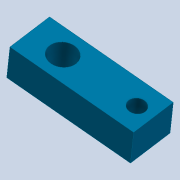
# Autodesk Inventor part: Part3_slider
Saved by Autodesk Inventor 2020 (Build 240168000, 168)
## iProperties
Created: 2019-05-16
Part Number: Part3_slider
Material: ABS Plastic
Document SubType Name: Modeling
Designer: kimhos
Density: 1.06 g/cm^3
Appearance: Sky Blue Medium
Author: kimhos
Autodesk Inventor part; units mm, degrees
ref_plane "YZ Plane" through (0, 0, 0) normal (1, 0, 0) x (0, 1, 0)
ref_plane "XZ Plane" through (0, 0, 0) normal (0, 1, 0) x (-1, 0, 0)
ref_plane "XY Plane" through (0, 0, 0) normal (0, 0, 1) x (1, 0, 0)
sketch "Sketch2" plane through (0, 0, 0) normal (0, 1, 0) x (-1, 0, 0)
  line L0 (1.35, 0) -> (1.35, -4.5)
  line L1 (-1.35, -1) -> (-1.35, 3)
  line L2 (-1.35, -4.5) -> (-1.35, 3)
  line L3 (-1.35, 3) -> (1.35, 3)
  line L4 (1.35, 3) -> (1.35, -4.5)
  line L5 (-1.35, -4.5) -> (1.35, -4.5)
  point P0 (0, 0)
  dimension "d8" = 1.35
  dimension "d11" = 4
  dimension "d24" = 7.5
  dimension "d62" = 2.7
  dimension "d63" = 2.7
  constraints: 12 end point, 2 vertical, 1 horizontal, 1 parallel
  measures "d8" distance of point (0, 0) L0.start
  measures "d11" distance of L1.start L1.end
  measures "d24" distance of L2.start L1.end
  measures "d62" distance of L1.end L3.end
  measures "d63" distance of L2.start L0.end
extrude "Extrusion1" add sketch "Sketch2" along normal mid plane 2
sketch "Sketch6" plane through (0, 1, 0) normal (0, 1, 0) x (1, 0, 0)
  line L0 (0, -3) -> (0, -1)
  circle A0 centre (0, -1) radius 0.8
  line L1 (0, -1) -> (-1.35, -1)
  line L2 (-1.35, 4.5) -> (-1.35, -3) projected
  point P0 (0, 0)
  dimension "d40" = 2
  dimension "d41" = 1.6
  dimension "d64" = 1.35
  constraints: 4 end point, 1 centre point, 1 coincident, 1 point on line, 1 vertical
  measures "d40" distance of L0.start L0.end
  measures "d41" diameter of A0
  measures "d64" distance of L1.start L1.end
hole "Hole3" at (0, 1, 1) direction (0, -1, 0) diameter 1.6 end through all
sketch "Sketch7" plane through (0, 1, 0) normal (0, 1, 0) x (1, 0, 0)
  line L0 (0, 4.5) -> (0, 3.5)
  circle A0 centre (0, 3.5) radius 0.5
  line L1 (0, 3.5) -> (0, -1)
  line L2 (0, 3.5) -> (0, 1)
  line L3 (0, 4.5) -> (0, 4)
  point P0 (0, 0)
  dimension "d50" = 1
  dimension "d49" = 1
  dimension "d51" = 4.5
  dimension "d52" = 2.5
  dimension "d53" = 0.5
  constraints: 8 end point, 2 vertical, 1 coincident, 1 point on line, 1 vertical alignment, 2 other
  measures "d49" distance of L0.start L0.end
  measures "d51" distance of L1.start L1.end
  measures "d52" distance of L1.start L2.end
  measures "d53" distance of L0.start L3.end
hole "Hole4" at (0, 1, -3.5) direction (0, -1, 0) diameter 1 end through all
body "Solid1"
